Autodesk Fusion 360 part; units mm, degrees
(part 7 of 8)
  spline S32 degree 5 poles (-4.5955, -17.2194) (-4.5901, -17.2152) (-4.5794, -17.2068) (-4.5635, -17.1938) (-4.543, -17.1757) (-4.5182, -17.1521) (-4.4941, -17.1278) (-4.4703, -17.103) (-4.4466, -17.078) (-4.4232, -17.0528) (-4.3998, -17.0274) (-4.3767, -17.0018) (-4.3538, -16.9759) (-4.3312, -16.9497) (-4.3089, -16.9231) (-4.2869, -16.8962) (-4.2651, -16.869) (-4.2435, -16.8416) (-4.2221, -16.814) (-4.2009, -16.7862) (-4.1798, -16.7583) (-4.1589, -16.7301) (-4.1383, -16.7018) (-4.1177, -16.6732) (-4.0974, -16.6444) (-4.0773, -16.6154) (-4.0574, -16.5863) (-4.0376, -16.5569) (-4.018, -16.5274) (-3.9985, -16.4977) (-3.9792, -16.4679) (-3.9601, -16.4379) (-3.9411, -16.4077) (-3.9223, -16.3774) (-3.9037, -16.3469) (-3.8852, -16.3163) (-3.8668, -16.2855) (-3.8486, -16.2545) (-3.8306, -16.2234) (-3.8127, -16.1922) (-3.795, -16.1608) (-3.7774, -16.1293) (-3.76, -16.0976) (-3.7427, -16.0658) (-3.7255, -16.0339) (-3.7085, -16.0018) (-3.6917, -15.9696) (-3.6749, -15.9373) (-3.6584, -15.9048) (-3.6419, -15.8722) (-3.6256, -15.8395) (-3.6095, -15.8066) (-3.5935, -15.7737) (-3.5776, -15.7406) (-3.5619, -15.7073) (-3.5463, -15.674) (-3.5308, -15.6406) (-3.5155, -15.607) (-3.5003, -15.5733) (-3.4853, -15.5395) (-3.4704, -15.5056) (-3.4556, -15.4715) (-3.4409, -15.4374) (-3.4264, -15.4031) (-3.412, -15.3688) (-3.3978, -15.3343) (-3.3837, -15.2997) (-3.3697, -15.265) (-3.3559, -15.2302) (-3.3422, -15.1953) (-3.3286, -15.1603) (-3.3178, -15.1322) (-3.3098, -15.1111) (-3.3045, -15.097) (-3.3018, -15.09) knots 0 0 0 0 0 0 0.01428571 0.02857143 0.04285714 0.05714286 0.07142857 0.08571429 0.1 0.11428571 0.12857143 0.14285714 0.15714286 0.17142857 0.18571429 0.2 0.21428571 0.22857143 0.24285714 0.25714286 0.27142857 0.28571429 0.3 0.31428571 0.32857143 0.34285714 0.35714286 0.37142857 0.38571429 0.4 0.41428571 0.42857143 0.44285714 0.45714286 0.47142857 0.48571429 0.5 0.51428571 0.52857143 0.54285714 0.55714286 0.57142857 0.58571429 0.6 0.61428571 0.62857143 0.64285714 0.65714286 0.67142857 0.68571429 0.7 0.71428571 0.72857143 0.74285714 0.75714286 0.77142857 0.78571429 0.8 0.81428571 0.82857143 0.84285714 0.85714286 0.87142857 0.88571429 0.9 0.91428571 0.92857143 0.94285714 0.95714286 0.97142857 0.98571429 1 1 1 1 1 1
  arc A66 (-3.3018, -15.09) -> (-3.8891, -14.427) centre (-17.3506, -26.9445) ccw
  spline S33 degree 5 poles (-3.8891, -14.427) (-3.8965, -14.4288) (-3.9111, -14.4324) (-3.933, -14.4378) (-3.9622, -14.4451) (-3.9986, -14.4544) (-4.0349, -14.4638) (-4.0711, -14.4733) (-4.1072, -14.483) (-4.1432, -14.4929) (-4.1792, -14.5028) (-4.215, -14.513) (-4.2508, -14.5233) (-4.2864, -14.5337) (-4.322, -14.5442) (-4.3575, -14.555) (-4.3929, -14.5658) (-4.4281, -14.5768) (-4.4633, -14.588) (-4.4984, -14.5993) (-4.5334, -14.6108) (-4.5682, -14.6224) (-4.603, -14.6342) (-4.6377, -14.6461) (-4.6722, -14.6581) (-4.7067, -14.6704) (-4.741, -14.6828) (-4.7752, -14.6953) (-4.8093, -14.708) (-4.8434, -14.7208) (-4.8772, -14.7339) (-4.911, -14.747) (-4.9447, -14.7604) (-4.9782, -14.7739) (-5.0116, -14.7875) (-5.0449, -14.8013) (-5.0781, -14.8153) (-5.1111, -14.8295) (-5.144, -14.8438) (-5.1768, -14.8583) (-5.2095, -14.873) (-5.242, -14.8878) (-5.2744, -14.9028) (-5.3066, -14.918) (-5.3387, -14.9334) (-5.3706, -14.949) (-5.4024, -14.9647) (-5.4341, -14.9806) (-5.4656, -14.9967) (-5.497, -15.013) (-5.5281, -15.0295) (-5.5592, -15.0462) (-5.59, -15.0631) (-5.6206, -15.0802) (-5.6511, -15.0975) (-5.6814, -15.1151) (-5.7116, -15.1328) (-5.7415, -15.1507) (-5.7713, -15.1688) (-5.8009, -15.1872) (-5.8303, -15.2058) (-5.8593, -15.2247) (-5.8881, -15.244) (-5.9166, -15.2636) (-5.9448, -15.2835) (-5.9728, -15.3036) (-6.0007, -15.3239) (-6.0283, -15.3443) (-6.0558, -15.3649) (-6.0829, -15.386) (-6.1093, -15.4078) (-6.1297, -15.4259) (-6.1445, -15.4401) (-6.1542, -15.4498) (-6.159, -15.4546) knots -1 -1 -1 -1 -1 -1 -0.98571429 -0.97142857 -0.95714286 -0.94285714 -0.92857143 -0.91428571 -0.9 -0.88571429 -0.87142857 -0.85714286 -0.84285714 -0.82857143 -0.81428571 -0.8 -0.78571429 -0.77142857 -0.75714286 -0.74285714 -0.72857143 -0.71428571 -0.7 -0.68571429 -0.67142857 -0.65714286 -0.64285714 -0.62857143 -0.61428571 -0.6 -0.58571429 -0.57142857 -0.55714286 -0.54285714 -0.52857143 -0.51428571 -0.5 -0.48571429 -0.47142857 -0.45714286 -0.44285714 -0.42857143 -0.41428571 -0.4 -0.38571429 -0.37142857 -0.35714286 -0.34285714 -0.32857143 -0.31428571 -0.3 -0.28571429 -0.27142857 -0.25714286 -0.24285714 -0.22857143 -0.21428571 -0.2 -0.18571429 -0.17142857 -0.15714286 -0.14285714 -0.12857143 -0.11428571 -0.1 -0.08571429 -0.07142857 -0.05714286 -0.04285714 -0.02857143 -0.01428571 0 0 0 0 0 0
  line L33 (-6.159, -15.4546) -> (-6.2327, -15.5301)
  arc A67 (-6.9279, -15.5497) -> (-6.2327, -15.5301) centre (-6.5904, -15.1808) ccw
  arc A68 (-6.9279, -15.5497) -> (-7.2953, -15.2243) centre (-17.3506, -26.9445) ccw
  arc A69 (-7.3596, -14.5317) -> (-7.2953, -15.2243) centre (-6.9697, -14.8448) ccw
  line L34 (-7.3596, -14.5317) -> (-7.2936, -14.4495)
  spline S34 degree 5 poles (-7.2936, -14.4495) (-7.2893, -14.4442) (-7.2808, -14.4334) (-7.2686, -14.417) (-7.253, -14.3945) (-7.2346, -14.3657) (-7.2169, -14.3363) (-7.1997, -14.3065) (-7.1828, -14.2766) (-7.1661, -14.2465) (-7.1495, -14.2162) (-7.1331, -14.1858) (-7.1171, -14.1552) (-7.1014, -14.1243) (-7.0861, -14.0932) (-7.0712, -14.0618) (-7.0565, -14.0302) (-7.0422, -13.9985) (-7.028, -13.9665) (-7.014, -13.9345) (-7.0003, -13.9023) (-6.9867, -13.87) (-6.9734, -13.8375) (-6.9604, -13.8048) (-6.9475, -13.772) (-6.9349, -13.7391) (-6.9225, -13.706) (-6.9103, -13.6728) (-6.8984, -13.6394) (-6.8866, -13.6059) (-6.875, -13.5724) (-6.8636, -13.5386) (-6.8524, -13.5048) (-6.8414, -13.4709) (-6.8306, -13.4368) (-6.8199, -13.4026) (-6.8095, -13.3683) (-6.7993, -13.3339) (-6.7892, -13.2994) (-6.7793, -13.2648) (-6.7696, -13.2301) (-6.7601, -13.1953) (-6.7507, -13.1604) (-6.7415, -13.1253) (-6.7325, -13.0902) (-6.7237, -13.055) (-6.715, -13.0197) (-6.7065, -12.9843) (-6.6982, -12.9488) (-6.6901, -12.9132) (-6.6821, -12.8776) (-6.6743, -12.8418) (-6.6666, -12.806) (-6.6591, -12.77) (-6.6518, -12.734) (-6.6446, -12.6979) (-6.6376, -12.6617) (-6.6308, -12.6255) (-6.6241, -12.5891) (-6.6176, -12.5527) (-6.6112, -12.5162) (-6.605, -12.4796) (-6.599, -12.443) (-6.5931, -12.4062) (-6.5873, -12.3694) (-6.5818, -12.3325) (-6.5763, -12.2956) (-6.5711, -12.2585) (-6.5659, -12.2214) (-6.561, -12.1843) (-6.5562, -12.147) (-6.5524, -12.1172) (-6.5497, -12.0948) (-6.5479, -12.0798) (-6.547, -12.0723) knots 0 0 0 0 0 0 0.01428571 0.02857143 0.04285714 0.05714286 0.07142857 0.08571429 0.1 0.11428571 0.12857143 0.14285714 0.15714286 0.17142857 0.18571429 0.2 0.21428571 0.22857143 0.24285714 0.25714286 0.27142857 0.28571429 0.3 0.31428571 0.32857143 0.34285714 0.35714286 0.37142857 0.38571429 0.4 0.41428571 0.42857143 0.44285714 0.45714286 0.47142857 0.48571429 0.5 0.51428571 0.52857143 0.54285714 0.55714286 0.57142857 0.58571429 0.6 0.61428571 0.62857143 0.64285714 0.65714286 0.67142857 0.68571429 0.7 0.71428571 0.72857143 0.74285714 0.75714286 0.77142857 0.78571429 0.8 0.81428571 0.82857143 0.84285714 0.85714286 0.87142857 0.88571429 0.9 0.91428571 0.92857143 0.94285714 0.95714286 0.97142857 0.98571429 1 1 1 1 1 1
  arc A70 (-6.547, -12.0723) -> (-7.2759, -11.5692) centre (-17.3506, -26.9445) ccw
  spline S35 degree 5 poles (-7.2759, -11.5692) (-7.2826, -11.5727) (-7.296, -11.5797) (-7.3159, -11.5902) (-7.3425, -11.6043) (-7.3756, -11.622) (-7.4086, -11.6398) (-7.4415, -11.6577) (-7.4743, -11.6758) (-7.5069, -11.694) (-7.5394, -11.7122) (-7.5718, -11.7307) (-7.604, -11.7492) (-7.6362, -11.7678) (-7.6682, -11.7866) (-7.7, -11.8055) (-7.7318, -11.8245) (-7.7634, -11.8437) (-7.7949, -11.8629) (-7.8262, -11.8823) (-7.8575, -11.9018) (-7.8885, -11.9214) (-7.9195, -11.9412) (-7.9503, -11.961) (-7.9809, -11.981) (-8.0115, -12.0011) (-8.0418, -12.0214) (-8.0721, -12.0417) (-8.1022, -12.0622) (-8.1321, -12.0829) (-8.1619, -12.1036) (-8.1915, -12.1245) (-8.221, -12.1455) (-8.2504, -12.1666) (-8.2795, -12.1879) (-8.3085, -12.2093) (-8.3374, -12.2308) (-8.3661, -12.2524) (-8.3946, -12.2742) (-8.423, -12.2961) (-8.4512, -12.3182) (-8.4792, -12.3404) (-8.507, -12.3627) (-8.5347, -12.3852) (-8.5622, -12.4078) (-8.5895, -12.4305) (-8.6166, -12.4534) (-8.6435, -12.4764) (-8.6703, -12.4996) (-8.6968, -12.5229) (-8.7231, -12.5464) (-8.7493, -12.57) (-8.7751, -12.5938) (-8.8008, -12.6178) (-8.8262, -12.6419) (-8.8515, -12.6662) (-8.8765, -12.6906) (-8.9013, -12.7152) (-8.9259, -12.7399) (-8.9502, -12.7648) (-8.9743, -12.7899) (-8.998, -12.8152) (-9.0213, -12.8408) (-9.0443, -12.8667) (-9.0669, -12.8928) (-9.0893, -12.919) (-9.1115, -12.9453) (-9.1335, -12.9718) (-9.1552, -12.9984) (-9.1764, -13.0253) (-9.1968, -13.0528) (-9.2123, -13.0753) (-9.2233, -13.0926) (-9.2304, -13.1043) (-9.2339, -13.1102) knots -1 -1 -1 -1 -1 -1 -0.98571429 -0.97142857 -0.95714286 -0.94285714 -0.92857143 -0.91428571 -0.9 -0.88571429 -0.87142857 -0.85714286 -0.84285714 -0.82857143 -0.81428571 -0.8 -0.78571429 -0.77142857 -0.75714286 -0.74285714 -0.72857143 -0.71428571 -0.7 -0.68571429 -0.67142857 -0.65714286 -0.64285714 -0.62857143 -0.61428571 -0.6 -0.58571429 -0.57142857 -0.55714286 -0.54285714 -0.52857143 -0.51428571 -0.5 -0.48571429 -0.47142857 -0.45714286 -0.44285714 -0.42857143 -0.41428571 -0.4 -0.38571429 -0.37142857 -0.35714286 -0.34285714 -0.32857143 -0.31428571 -0.3 -0.28571429 -0.27142857 -0.25714286 -0.24285714 -0.22857143 -0.21428571 -0.2 -0.18571429 -0.17142857 -0.15714286 -0.14285714 -0.12857143 -0.11428571 -0.1 -0.08571429 -0.07142857 -0.05714286 -0.04285714 -0.02857143 -0.01428571 0 0 0 0 0 0
  line L35 (-9.2339, -13.1102) -> (-9.2874, -13.2011)
  arc A71 (-9.9577, -13.3865) -> (-9.2874, -13.2011) centre (-9.7183, -12.9475) ccw
  arc A72 (-9.9577, -13.3865) -> (-10.3923, -13.1584) centre (-17.3506, -26.9445) ccw
  arc A73 (-10.6205, -12.5014) -> (-10.3923, -13.1584) centre (-10.167, -12.7121) ccw
  line L36 (-10.6205, -12.5014) -> (-10.576, -12.4058)
  spline S36 degree 5 poles (-10.576, -12.4058) (-10.5732, -12.3996) (-10.5675, -12.3871) (-10.5596, -12.3682) (-10.5498, -12.3427) (-10.5389, -12.3103) (-10.5288, -12.2775) (-10.5192, -12.2445) (-10.5099, -12.2114) (-10.5008, -12.1781) (-10.492, -12.1448) (-10.4834, -12.1114) (-10.4751, -12.0778) (-10.4673, -12.0441) (-10.4599, -12.0102) (-10.4529, -11.9761) (-10.4463, -11.942) (-10.4399, -11.9077) (-10.4338, -11.8733) (-10.4279, -11.8388) (-10.4222, -11.8043) (-10.4168, -11.7696) (-10.4117, -11.7349) (-10.4068, -11.7001) (-10.4022, -11.6652) (-10.3978, -11.6302) (-10.3937, -11.5951) (-10.3899, -11.5599) (-10.3862, -11.5246) (-10.3828, -11.4893) (-10.3795, -11.4539) (-10.3765, -11.4185) (-10.3738, -11.383) (-10.3712, -11.3474) (-10.3689, -11.3117) (-10.3667, -11.276) (-10.3648, -11.2402) (-10.3631, -11.2043) (-10.3616, -11.1684) (-10.3602, -11.1324) (-10.3591, -11.0964) (-10.3582, -11.0603) (-10.3575, -11.0242) (-10.3569, -10.988) (-10.3566, -10.9517) (-10.3564, -10.9154) (-10.3565, -10.8791) (-10.3567, -10.8427) (-10.3571, -10.8062) (-10.3577, -10.7697) (-10.3585, -10.7332) (-10.3595, -10.6966) (-10.3606, -10.6599) (-10.362, -10.6233) (-10.3635, -10.5865) (-10.3651, -10.5498) (-10.367, -10.513) (-10.369, -10.4761) (-10.3713, -10.4392) (-10.3736, -10.4023) (-10.3762, -10.3653) (-10.3789, -10.3283) (-10.3818, -10.2913) (-10.3849, -10.2542) (-10.3881, -10.2171) (-10.3915, -10.18) (-10.3951, -10.1428) (-10.3989, -10.1056) (-10.4028, -10.0683) (-10.4069, -10.0311) (-10.4111, -9.9938) (-10.4146, -9.9639) (-10.4173, -9.9415) (-10.4192, -9.9265) (-10.4201, -9.919) knots 0 0 0 0 0 0 0.01428571 0.02857143 0.04285714 0.05714286 0.07142857 0.08571429 0.1 0.11428571 0.12857143 0.14285714 0.15714286 0.17142857 0.18571429 0.2 0.21428571 0.22857143 0.24285714 0.25714286 0.27142857 0.28571429 0.3 0.31428571 0.32857143 0.34285714 0.35714286 0.37142857 0.38571429 0.4 0.41428571 0.42857143 0.44285714 0.45714286 0.47142857 0.48571429 0.5 0.51428571 0.52857143 0.54285714 0.55714286 0.57142857 0.58571429 0.6 0.61428571 0.62857143 0.64285714 0.65714286 0.67142857 0.68571429 0.7 0.71428571 0.72857143 0.74285714 0.75714286 0.77142857 0.78571429 0.8 0.81428571 0.82857143 0.84285714 0.85714286 0.87142857 0.88571429 0.9 0.91428571 0.92857143 0.94285714 0.95714286 0.97142857 0.98571429 1 1 1 1 1 1
  arc A74 (-10.4201, -9.919) -> (-11.2482, -9.605) centre (-17.3506, -26.9445) ccw
  spline S37 degree 5 poles (-11.2482, -9.605) (-11.2539, -9.61) (-11.2652, -9.6199) (-11.2821, -9.6349) (-11.3045, -9.6549) (-11.3324, -9.68) (-11.3602, -9.7052) (-11.3878, -9.7305) (-11.4153, -9.7559) (-11.4426, -9.7813) (-11.4698, -9.8069) (-11.4968, -9.8325) (-11.5237, -9.8582) (-11.5505, -9.884) (-11.577, -9.9099) (-11.6035, -9.9359) (-11.6297, -9.962) (-11.6559, -9.9881) (-11.6818, -10.0143) (-11.7076, -10.0406) (-11.7333, -10.067) (-11.7587, -10.0935) (-11.7841, -10.1201) (-11.8092, -10.1468) (-11.8342, -10.1735) (-11.859, -10.2004) (-11.8837, -10.2273) (-11.9082, -10.2543) (-11.9325, -10.2814) (-11.9566, -10.3086) (-11.9806, -10.3358) (-12.0043, -10.3632) (-12.0279, -10.3906) (-12.0514, -10.4182) (-12.0746, -10.4458) (-12.0977, -10.4735) (-12.1205, -10.5013) (-12.1432, -10.5292) (-12.1657, -10.5572) (-12.188, -10.5853) (-12.2101, -10.6134) (-12.232, -10.6417) (-12.2537, -10.67) (-12.2751, -10.6984) (-12.2964, -10.727) (-12.3175, -10.7556) (-12.3383, -10.7843) (-12.359, -10.8131) (-12.3794, -10.842) (-12.3996, -10.871) (-12.4195, -10.9001) (-12.4392, -10.9293) (-12.4587, -10.9586) (-12.4778, -10.988) (-12.4968, -11.0175) (-12.5155, -11.0471) (-12.5339, -11.0768) (-12.5521, -11.1066) (-12.5701, -11.1365) (-12.5878, -11.1665) (-12.6051, -11.1966) (-12.622, -11.2269) (-12.6386, -11.2573) (-12.6547, -11.2879) (-12.6704, -11.3186) (-12.6858, -11.3495) (-12.7011, -11.3804) (-12.7161, -11.4113) (-12.7308, -11.4424) (-12.745, -11.4736) (-12.7583, -11.5051) (-12.7679, -11.5307) (-12.7745, -11.5501) (-12.7786, -11.5632) (-12.7805, -11.5697) knots -1 -1 -1 -1 -1 -1 -0.98571429 -0.97142857 -0.95714286 -0.94285714 -0.92857143 -0.91428571 -0.9 -0.88571429 -0.87142857 -0.85714286 -0.84285714 -0.82857143 -0.81428571 -0.8 -0.78571429 -0.77142857 -0.75714286 -0.74285714 -0.72857143 -0.71428571 -0.7 -0.68571429 -0.67142857 -0.65714286 -0.64285714 -0.62857143 -0.61428571 -0.6 -0.58571429 -0.57142857 -0.55714286 -0.54285714 -0.52857143 -0.51428571 -0.5 -0.48571429 -0.47142857 -0.45714286 -0.44285714 -0.42857143 -0.41428571 -0.4 -0.38571429 -0.37142857 -0.35714286 -0.34285714 -0.32857143 -0.31428571 -0.3 -0.28571429 -0.27142857 -0.25714286 -0.24285714 -0.22857143 -0.21428571 -0.2 -0.18571429 -0.17142857 -0.15714286 -0.14285714 -0.12857143 -0.11428571 -0.1 -0.08571429 -0.07142857 -0.05714286 -0.04285714 -0.02857143 -0.01428571 0 0 0 0 0 0
  line L37 (-12.7805, -11.5697) -> (-12.8107, -11.6708)
  arc A75 (-13.4171, -12.0112) -> (-12.8107, -11.6708) centre (-13.2898, -11.5277) ccw
  arc A76 (-13.4171, -12.0112) -> (-13.8937, -11.8938) centre (-17.3506, -26.9445) ccw
  arc A77 (-14.2725, -11.3105) -> (-13.8937, -11.8938) centre (-13.7818, -11.4065) ccw
  line L38 (-14.2725, -11.3105) -> (-14.2522, -11.207)
  spline S38 degree 5 poles (-14.2522, -11.207) (-14.2509, -11.2003) (-14.2485, -11.1868) (-14.2453, -11.1666) (-14.2419, -11.1394) (-14.239, -11.1054) (-14.237, -11.0711) (-14.2356, -11.0368) (-14.2346, -11.0024) (-14.2337, -10.968) (-14.2331, -10.9335) (-14.2327, -10.899) (-14.2328, -10.8644) (-14.2332, -10.8298) (-14.2342, -10.7951) (-14.2355, -10.7604) (-14.2372, -10.7256) (-14.2393, -10.6908) (-14.2415, -10.6559) (-14.2441, -10.6211) (-14.2469, -10.5862) (-14.2499, -10.5512) (-14.2532, -10.5163) (-14.2568, -10.4813) (-14.2607, -10.4463) (-14.2648, -10.4113) (-14.2692, -10.3762) (-14.2739, -10.3411) (-14.2788, -10.306) (-14.2839, -10.2709) (-14.2892, -10.2358) (-14.2948, -10.2006) (-14.3006, -10.1655) (-14.3067, -10.1303) (-14.3129, -10.0951) (-14.3194, -10.0599) (-14.3261, -10.0247) (-14.333, -9.9895) (-14.3401, -9.9542) (-14.3474, -9.919) (-14.355, -9.8837) (-14.3627, -9.8485) (-14.3707, -9.8132) (-14.3788, -9.778) (-14.3871, -9.7427) (-14.3957, -9.7074) (-14.4044, -9.6721) (-14.4134, -9.6368) (-14.4225, -9.6015) (-14.4318, -9.5662) (-14.4413, -9.5309) (-14.451, -9.4956) (-14.4609, -9.4603) (-14.471, -9.425) (-14.4812, -9.3897) (-14.4916, -9.3544) (-14.5023, -9.3192) (-14.513, -9.2839) (-14.524, -9.2486) (-14.5352, -9.2133) (-14.5465, -9.178) (-14.558, -9.1427) (-14.5697, -9.1075) (-14.5816, -9.0722) (-14.5936, -9.0369) (-14.6058, -9.0017) (-14.6182, -8.9665) (-14.6307, -8.9312) (-14.6434, -8.896) (-14.6563, -8.8608) (-14.6693, -8.8256) (-14.6799, -8.7974) (-14.6879, -8.7763) (-14.6933, -8.7622) (-14.696, -8.7552) knots 0 0 0 0 0 0 0.01428571 0.02857143 0.04285714 0.05714286 0.07142857 0.08571429 0.1 0.11428571 0.12857143 0.14285714 0.15714286 0.17142857 0.18571429 0.2 0.21428571 0.22857143 0.24285714 0.25714286 0.27142857 0.28571429 0.3 0.31428571 0.32857143 0.34285714 0.35714286 0.37142857 0.38571429 0.4 0.41428571 0.42857143 0.44285714 0.45714286 0.47142857 0.48571429 0.5 0.51428571 0.52857143 0.54285714 0.55714286 0.57142857 0.58571429 0.6 0.61428571 0.62857143 0.64285714 0.65714286 0.67142857 0.68571429 0.7 0.71428571 0.72857143 0.74285714 0.75714286 0.77142857 0.78571429 0.8 0.81428571 0.82857143 0.84285714 0.85714286 0.87142857 0.88571429 0.9 0.91428571 0.92857143 0.94285714 0.95714286 0.97142857 0.98571429 1 1 1 1 1 1
  arc A78 (-14.696, -8.7552) -> (-15.5752, -8.6484) centre (-17.3506, -26.9445) ccw
  spline S39 degree 5 poles (-15.5752, -8.6484) (-15.5795, -8.6546) (-15.588, -8.667) (-15.6009, -8.6856) (-15.6179, -8.7104) (-15.639, -8.7415) (-15.6599, -8.7726) (-15.6807, -8.8037) (-15.7013, -8.8349) (-15.7217, -8.8662) (-15.742, -8.8975) (-15.7621, -8.9289) (-15.7821, -8.9603) (-15.8018, -8.9917) (-15.8215, -9.0232) (-15.8409, -9.0547) (-15.8602, -9.0863) (-15.8793, -9.118) (-15.8982, -9.1497) (-15.9169, -9.1814) (-15.9355, -9.2132) (-15.9539, -9.245) (-15.9721, -9.2768) (-15.9902, -9.3087) (-16.008, -9.3407) (-16.0257, -9.3727) (-16.0432, -9.4047) (-16.0605, -9.4368) (-16.0776, -9.4689) (-16.0946, -9.5011) (-16.1113, -9.5333) (-16.1279, -9.5656) (-16.1442, -9.5979) (-16.1604, -9.6302) (-16.1763, -9.6626) (-16.1921, -9.695) (-16.2076, -9.7275) (-16.223, -9.76) (-16.2381, -9.7925) (-16.253, -9.8251) (-16.2677, -9.8578) (-16.2822, -9.8904) (-16.2965, -9.9231) (-16.3106, -9.9559) (-16.3244, -9.9887) (-16.338, -10.0215) (-16.3513, -10.0544) (-16.3645, -10.0873) (-16.3774, -10.1202) (-16.3901, -10.1532) (-16.4025, -10.1862) (-16.4146, -10.2193) (-16.4265, -10.2524) (-16.4381, -10.2855) (-16.4494, -10.3187) (-16.4604, -10.3519) (-16.4712, -10.3852) (-16.4818, -10.4185) (-16.4921, -10.4518) (-16.5021, -10.4852) (-16.5117, -10.5186) (-16.5209, -10.552) (-16.5297, -10.5855) (-16.538, -10.6191) (-16.5459, -10.6527) (-16.5535, -10.6863) (-16.5609, -10.7199) (-16.5681, -10.7536) (-16.575, -10.7872) (-16.5813, -10.8209) (-16.5866, -10.8548) (-16.5898, -10.8819) (-16.5916, -10.9023) (-16.5924, -10.916) (-16.5927, -10.9228) knots -1 -1 -1 -1 -1 -1 -0.98571429 -0.97142857 -0.95714286 -0.94285714 -0.92857143 -0.91428571 -0.9 -0.88571429 -0.87142857 -0.85714286 -0.84285714 -0.82857143 -0.81428571 -0.8 -0.78571429 -0.77142857 -0.75714286 -0.74285714 -0.72857143 -0.71428571 -0.7 -0.68571429 -0.67142857 -0.65714286 -0.64285714 -0.62857143 -0.61428571 -0.6 -0.58571429 -0.57142857 -0.55714286 -0.54285714 -0.52857143 -0.51428571 -0.5 -0.48571429 -0.47142857 -0.45714286 -0.44285714 -0.42857143 -0.41428571 -0.4 -0.38571429 -0.37142857 -0.35714286 -0.34285714 -0.32857143 -0.31428571 -0.3 -0.28571429 -0.27142857 -0.25714286 -0.24285714 -0.22857143 -0.21428571 -0.2 -0.18571429 -0.17142857 -0.15714286 -0.14285714 -0.12857143 -0.11428571 -0.1 -0.08571429 -0.07142857 -0.05714286 -0.04285714 -0.02857143 -0.01428571 0 0 0 0 0 0
  line L39 (-16.5927, -10.9228) -> (-16.5978, -11.0281)
  arc A79 (-17.1052, -11.5038) -> (-16.5978, -11.0281) centre (-17.0973, -11.0039) ccw
  arc A80 (-17.1052, -11.5038) -> (-17.596, -11.5038) centre (-17.3506, -26.9445) ccw
  arc A81 (-18.1034, -11.0281) -> (-17.596, -11.5038) centre (-17.604, -11.0039) ccw
  line L40 (-18.1034, -11.0281) -> (-18.1085, -10.9228)
  spline S40 degree 5 poles (-18.1085, -10.9228) (-18.1088, -10.916) (-18.1097, -10.9023) (-18.1114, -10.8819) (-18.1146, -10.8548) (-18.12, -10.8209) (-18.1262, -10.7872) (-18.1331, -10.7536) (-18.1403, -10.7199) (-18.1477, -10.6863) (-18.1553, -10.6527) (-18.1633, -10.6191) (-18.1716, -10.5855) (-18.1803, -10.552) (-18.1895, -10.5186) (-18.1992, -10.4852) (-18.2091, -10.4518) (-18.2194, -10.4185) (-18.23, -10.3852) (-18.2408, -10.3519) (-18.2518, -10.3187) (-18.2632, -10.2855) (-18.2747, -10.2524) (-18.2866, -10.2193) (-18.2988, -10.1862) (-18.3112, -10.1532) (-18.3238, -10.1202) (-18.3367, -10.0873) (-18.3499, -10.0544) (-18.3633, -10.0215) (-18.3769, -9.9887) (-18.3907, -9.9559) (-18.4047, -9.9231) (-18.419, -9.8904) (-18.4335, -9.8578) (-18.4482, -9.8251) (-18.4631, -9.7925) (-18.4783, -9.76) (-18.4936, -9.7275) (-18.5092, -9.695) (-18.5249, -9.6626) (-18.5409, -9.6302) (-18.557, -9.5979) (-18.5734, -9.5656) (-18.5899, -9.5333) (-18.6067, -9.5011) (-18.6236, -9.4689) (-18.6407, -9.4368) (-18.658, -9.4047) (-18.6755, -9.3727) (-18.6932, -9.3407) (-18.711, -9.3087) (-18.7291, -9.2768) (-18.7473, -9.245) (-18.7657, -9.2132) (-18.7843, -9.1814) (-18.803, -9.1497) (-18.822, -9.118) (-18.8411, -9.0863) (-18.8603, -9.0547) (-18.8798, -9.0232) (-18.8994, -8.9917) (-18.9192, -8.9603) (-18.9391, -8.9289) (-18.9592, -8.8975) (-18.9795, -8.8662) (-19, -8.8349) (-19.0206, -8.8037) (-19.0414, -8.7726) (-19.0623, -8.7415) (-19.0834, -8.7104) (-19.1004, -8.6856) (-19.1132, -8.667) (-19.1218, -8.6546) (-19.1261, -8.6484) knots 0 0 0 0 0 0 0.01428571 0.02857143 0.04285714 0.05714286 0.07142857 0.08571429 0.1 0.11428571 0.12857143 0.14285714 0.15714286 0.17142857 0.18571429 0.2 0.21428571 0.22857143 0.24285714 0.25714286 0.27142857 0.28571429 0.3 0.31428571 0.32857143 0.34285714 0.35714286 0.37142857 0.38571429 0.4 0.41428571 0.42857143 0.44285714 0.45714286 0.47142857 0.48571429 0.5 0.51428571 0.52857143 0.54285714 0.55714286 0.57142857 0.58571429 0.6 0.61428571 0.62857143 0.64285714 0.65714286 0.67142857 0.68571429 0.7 0.71428571 0.72857143 0.74285714 0.75714286 0.77142857 0.78571429 0.8 0.81428571 0.82857143 0.84285714 0.85714286 0.87142857 0.88571429 0.9 0.91428571 0.92857143 0.94285714 0.95714286 0.97142857 0.98571429 1 1 1 1 1 1
  arc A82 (-19.1261, -8.6484) -> (-20.0053, -8.7552) centre (-17.3506, -26.9445) ccw
  spline S41 degree 5 poles (-20.0053, -8.7552) (-20.008, -8.7622) (-20.0133, -8.7763) (-20.0213, -8.7974) (-20.0319, -8.8256) (-20.045, -8.8608) (-20.0578, -8.896) (-20.0705, -8.9312) (-20.0831, -8.9665) (-20.0955, -9.0017) (-20.1077, -9.0369) (-20.1197, -9.0722) (-20.1315, -9.1075) (-20.1432, -9.1427) (-20.1547, -9.178) (-20.1661, -9.2133) (-20.1772, -9.2486) (-20.1882, -9.2839) (-20.199, -9.3192) (-20.2096, -9.3544) (-20.22, -9.3897) (-20.2303, -9.425) (-20.2404, -9.4603) (-20.2502, -9.4956) (-20.2599, -9.5309) (-20.2694, -9.5662) (-20.2787, -9.6015) (-20.2879, -9.6368) (-20.2968, -9.6721) (-20.3055, -9.7074) (-20.3141, -9.7427) (-20.3224, -9.778) (-20.3306, -9.8132) (-20.3385, -9.8485) (-20.3463, -9.8837) (-20.3538, -9.919) (-20.3611, -9.9542) (-20.3682, -9.9895) (-20.3752, -10.0247) (-20.3819, -10.0599) (-20.3883, -10.0951) (-20.3946, -10.1303) (-20.4006, -10.1655) (-20.4064, -10.2006) (-20.412, -10.2358) (-20.4173, -10.2709) (-20.4225, -10.306) (-20.4273, -10.3411) (-20.432, -10.3762) (-20.4364, -10.4113) (-20.4406, -10.4463) (-20.4444, -10.4813) (-20.448, -10.5163) (-20.4513, -10.5512) (-20.4544, -10.5862) (-20.4572, -10.6211) (-20.4597, -10.6559) (-20.462, -10.6908) (-20.464, -10.7256) (-20.4657, -10.7604) (-20.4671, -10.7951) (-20.468, -10.8298) (-20.4685, -10.8644) (-20.4685, -10.899) (-20.4682, -10.9335) (-20.4675, -10.968) (-20.4667, -11.0024) (-20.4656, -11.0368) (-20.4642, -11.0711) (-20.4622, -11.1054) (-20.4593, -11.1394) (-20.456, -11.1666) (-20.4528, -11.1868) (-20.4503, -11.2003) (-20.449, -11.207) knots -1 -1 -1 -1 -1 -1 -0.98571429 -0.97142857 -0.95714286 -0.94285714 -0.92857143 -0.91428571 -0.9 -0.88571429 -0.87142857 -0.85714286 -0.84285714 -0.82857143 -0.81428571 -0.8 -0.78571429 -0.77142857 -0.75714286 -0.74285714 -0.72857143 -0.71428571 -0.7 -0.68571429 -0.67142857 -0.65714286 -0.64285714 -0.62857143 -0.61428571 -0.6 -0.58571429 -0.57142857 -0.55714286 -0.54285714 -0.52857143 -0.51428571 -0.5 -0.48571429 -0.47142857 -0.45714286 -0.44285714 -0.42857143 -0.41428571 -0.4 -0.38571429 -0.37142857 -0.35714286 -0.34285714 -0.32857143 -0.31428571 -0.3 -0.28571429 -0.27142857 -0.25714286 -0.24285714 -0.22857143 -0.21428571 -0.2 -0.18571429 -0.17142857 -0.15714286 -0.14285714 -0.12857143 -0.11428571 -0.1 -0.08571429 -0.07142857 -0.05714286 -0.04285714 -0.02857143 -0.01428571 0 0 0 0 0 0
  line L41 (-20.449, -11.207) -> (-20.4288, -11.3105)
  arc A83 (-20.8075, -11.8938) -> (-20.4288, -11.3105) centre (-20.9195, -11.4065) ccw
  arc A84 (-20.8075, -11.8938) -> (-21.2841, -12.0112) centre (-17.3506, -26.9445) ccw
  arc A85 (-21.8906, -11.6708) -> (-21.2841, -12.0112) centre (-21.4115, -11.5277) ccw
  line L42 (-21.8906, -11.6708) -> (-21.9207, -11.5697)
  spline S42 degree 5 poles (-21.9207, -11.5697) (-21.9227, -11.5632) (-21.9267, -11.5501) (-21.9333, -11.5307) (-21.943, -11.5051) (-21.9562, -11.4736) (-21.9704, -11.4424) (-21.9851, -11.4113) (-22.0001, -11.3804) (-22.0154, -11.3495) (-22.0308, -11.3186) (-22.0466, -11.2879) (-22.0627, -11.2573) (-22.0792, -11.2269) (-22.0961, -11.1966) (-22.1135, -11.1665) (-22.1312, -11.1365) (-22.1491, -11.1066) (-22.1673, -11.0768) (-22.1858, -11.0471) (-22.2045, -11.0175) (-22.2234, -10.988) (-22.2426, -10.9586) (-22.262, -10.9293) (-22.2817, -10.9001) (-22.3017, -10.871) (-22.3219, -10.842) (-22.3423, -10.8131) (-22.3629, -10.7843) (-22.3838, -10.7556) (-22.4048, -10.727) (-22.4261, -10.6984) (-22.4476, -10.67) (-22.4693, -10.6417) (-22.4912, -10.6134) (-22.5132, -10.5853) (-22.5355, -10.5572) (-22.558, -10.5292) (-22.5807, -10.5013) (-22.6036, -10.4735) (-22.6266, -10.4458) (-22.6499, -10.4182) (-22.6733, -10.3906) (-22.6969, -10.3632) (-22.7207, -10.3358) (-22.7446, -10.3086) (-22.7688, -10.2814) (-22.7931, -10.2543) (-22.8176, -10.2273) (-22.8422, -10.2004) (-22.867, -10.1735) (-22.892, -10.1468) (-22.9172, -10.1201) (-22.9425, -10.0935) (-22.968, -10.067) (-22.9936, -10.0406) (-23.0194, -10.0143) (-23.0454, -9.9881) (-23.0715, -9.962) (-23.0978, -9.9359) (-23.1242, -9.9099) (-23.1508, -9.884) (-23.1775, -9.8582) (-23.2044, -9.8325) (-23.2314, -9.8069) (-23.2586, -9.7813) (-23.2859, -9.7559) (-23.3134, -9.7305) (-23.341, -9.7052) (-23.3688, -9.68) (-23.3967, -9.6549) (-23.4192, -9.6349) (-23.4361, -9.6199) (-23.4474, -9.61) (-23.453, -9.605) knots 0 0 0 0 0 0 0.01428571 0.02857143 0.04285714 0.05714286 0.07142857 0.08571429 0.1 0.11428571 0.12857143 0.14285714 0.15714286 0.17142857 0.18571429 0.2 0.21428571 0.22857143 0.24285714 0.25714286 0.27142857 0.28571429 0.3 0.31428571 0.32857143 0.34285714 0.35714286 0.37142857 0.38571429 0.4 0.41428571 0.42857143 0.44285714 0.45714286 0.47142857 0.48571429 0.5 0.51428571 0.52857143 0.54285714 0.55714286 0.57142857 0.58571429 0.6 0.61428571 0.62857143 0.64285714 0.65714286 0.67142857 0.68571429 0.7 0.71428571 0.72857143 0.74285714 0.75714286 0.77142857 0.78571429 0.8 0.81428571 0.82857143 0.84285714 0.85714286 0.87142857 0.88571429 0.9 0.91428571 0.92857143 0.94285714 0.95714286 0.97142857 0.98571429 1 1 1 1 1 1
  arc A86 (-23.453, -9.605) -> (-24.2811, -9.919) centre (-17.3506, -26.9445) ccw
  spline S43 degree 5 poles (-24.2811, -9.919) (-24.2821, -9.9265) (-24.2839, -9.9415) (-24.2866, -9.9639) (-24.2901, -9.9938) (-24.2944, -10.0311) (-24.2985, -10.0683) (-24.3024, -10.1056) (-24.3061, -10.1428) (-24.3097, -10.18) (-24.3131, -10.2171) (-24.3163, -10.2542) (-24.3194, -10.2913) (-24.3223, -10.3283) (-24.325, -10.3653) (-24.3276, -10.4023) (-24.33, -10.4392) (-24.3322, -10.4761) (-24.3342, -10.513) (-24.3361, -10.5498) (-24.3378, -10.5865) (-24.3393, -10.6233) (-24.3406, -10.6599) (-24.3418, -10.6966) (-24.3427, -10.7332) (-24.3435, -10.7697) (-24.3441, -10.8062) (-24.3445, -10.8427) (-24.3447, -10.8791) (-24.3448, -10.9154) (-24.3446, -10.9517) (-24.3443, -10.988) (-24.3438, -11.0242) (-24.343, -11.0603) (-24.3421, -11.0964) (-24.341, -11.1324) (-24.3397, -11.1684) (-24.3382, -11.2043) (-24.3364, -11.2402) (-24.3345, -11.276) (-24.3324, -11.3117) (-24.33, -11.3474) (-24.3275, -11.383) (-24.3247, -11.4185) (-24.3217, -11.4539) (-24.3185, -11.4893) (-24.315, -11.5246) (-24.3114, -11.5599) (-24.3075, -11.5951) (-24.3034, -11.6302) (-24.299, -11.6652) (-24.2944, -11.7001) (-24.2896, -11.7349) (-24.2844, -11.7696) (-24.279, -11.8043) (-24.2734, -11.8388) (-24.2675, -11.8733) (-24.2613, -11.9077) (-24.255, -11.942) (-24.2483, -11.9761) (-24.2413, -12.0102) (-24.2339, -12.0441) (-24.2261, -12.0778) (-24.2179, -12.1114) (-24.2093, -12.1448) (-24.2004, -12.1781) (-24.1913, -12.2114) (-24.1821, -12.2445) (-24.1725, -12.2775) (-24.1624, -12.3103) (-24.1514, -12.3427) (-24.1416, -12.3682) (-24.1337, -12.3871) (-24.1281, -12.3996) (-24.1252, -12.4058) knots -1 -1 -1 -1 -1 -1 -0.98571429 -0.97142857 -0.95714286 -0.94285714 -0.92857143 -0.91428571 -0.9 -0.88571429 -0.87142857 -0.85714286 -0.84285714 -0.82857143 -0.81428571 -0.8 -0.78571429 -0.77142857 -0.75714286 -0.74285714 -0.72857143 -0.71428571 -0.7 -0.68571429 -0.67142857 -0.65714286 -0.64285714 -0.62857143 -0.61428571 -0.6 -0.58571429 -0.57142857 -0.55714286 -0.54285714 -0.52857143 -0.51428571 -0.5 -0.48571429 -0.47142857 -0.45714286 -0.44285714 -0.42857143 -0.41428571 -0.4 -0.38571429 -0.37142857 -0.35714286 -0.34285714 -0.32857143 -0.31428571 -0.3 -0.28571429 -0.27142857 -0.25714286 -0.24285714 -0.22857143 -0.21428571 -0.2 -0.18571429 -0.17142857 -0.15714286 -0.14285714 -0.12857143 -0.11428571 -0.1 -0.08571429 -0.07142857 -0.05714286 -0.04285714 -0.02857143 -0.01428571 0 0 0 0 0 0
  line L43 (-24.1252, -12.4058) -> (-24.0808, -12.5014)
  arc A87 (-24.3089, -13.1584) -> (-24.0808, -12.5014) centre (-24.5342, -12.7121) ccw
  arc A88 (-24.3089, -13.1584) -> (-24.7436, -13.3865) centre (-17.3506, -26.9445) ccw
  arc A89 (-25.4139, -13.2011) -> (-24.7436, -13.3865) centre (-24.9829, -12.9475) ccw
  line L44 (-25.4139, -13.2011) -> (-25.4673, -13.1102)
  spline S44 degree 5 poles (-25.4673, -13.1102) (-25.4708, -13.1043) (-25.4779, -13.0926) (-25.4889, -13.0753) (-25.5044, -13.0528) (-25.5248, -13.0253) (-25.5461, -12.9984) (-25.5678, -12.9718) (-25.5898, -12.9453) (-25.612, -12.919) (-25.6344, -12.8928) (-25.657, -12.8667) (-25.6799, -12.8408) (-25.7033, -12.8152) (-25.7269, -12.7899) (-25.751, -12.7648) (-25.7753, -12.7399) (-25.7999, -12.7152) (-25.8248, -12.6906) (-25.8498, -12.6662) (-25.875, -12.6419) (-25.9004, -12.6178) (-25.9261, -12.5938) (-25.952, -12.57) (-25.9781, -12.5464) (-26.0044, -12.5229) (-26.031, -12.4996) (-26.0577, -12.4764) (-26.0847, -12.4534) (-26.1118, -12.4305) (-26.1391, -12.4078) (-26.1665, -12.3852) (-26.1942, -12.3627) (-26.222, -12.3404) (-26.2501, -12.3182) (-26.2783, -12.2961) (-26.3066, -12.2742) (-26.3351, -12.2524) (-26.3638, -12.2308) (-26.3927, -12.2093) (-26.4217, -12.1879) (-26.4509, -12.1666) (-26.4802, -12.1455) (-26.5097, -12.1245) (-26.5393, -12.1036) (-26.5691, -12.0829) (-26.5991, -12.0622) (-26.6292, -12.0417) (-26.6594, -12.0214) (-26.6898, -12.0011) (-26.7203, -11.981) (-26.751, -11.961) (-26.7818, -11.9412) (-26.8127, -11.9214) (-26.8438, -11.9018) (-26.875, -11.8823) (-26.9063, -11.8629) (-26.9378, -11.8437) (-26.9694, -11.8245) (-27.0012, -11.8055) (-27.0331, -11.7866) (-27.0651, -11.7678) (-27.0972, -11.7492) (-27.1295, -11.7307) (-27.1618, -11.7122) (-27.1943, -11.694) (-27.227, -11.6758) (-27.2597, -11.6577) (-27.2926, -11.6398) (-27.3256, -11.622) (-27.3587, -11.6043) (-27.3853, -11.5902) (-27.4053, -11.5797) (-27.4186, -11.5727) (-27.4253, -11.5692) knots 0 0 0 0 0 0 0.01428571 0.02857143 0.04285714 0.05714286 0.07142857 0.08571429 0.1 0.11428571 0.12857143 0.14285714 0.15714286 0.17142857 0.18571429 0.2 0.21428571 0.22857143 0.24285714 0.25714286 0.27142857 0.28571429 0.3 0.31428571 0.32857143 0.34285714 0.35714286 0.37142857 0.38571429 0.4 0.41428571 0.42857143 0.44285714 0.45714286 0.47142857 0.48571429 0.5 0.51428571 0.52857143 0.54285714 0.55714286 0.57142857 0.58571429 0.6 0.61428571 0.62857143 0.64285714 0.65714286 0.67142857 0.68571429 0.7 0.71428571 0.72857143 0.74285714 0.75714286 0.77142857 0.78571429 0.8 0.81428571 0.82857143 0.84285714 0.85714286 0.87142857 0.88571429 0.9 0.91428571 0.92857143 0.94285714 0.95714286 0.97142857 0.98571429 1 1 1 1 1 1
  arc A90 (-27.4253, -11.5692) -> (-28.1542, -12.0723) centre (-17.3506, -26.9445) ccw
  spline S45 degree 5 poles (-28.1542, -12.0723) (-28.1533, -12.0798) (-28.1515, -12.0948) (-28.1488, -12.1172) (-28.1451, -12.147) (-28.1403, -12.1843) (-28.1353, -12.2214) (-28.1302, -12.2585) (-28.1249, -12.2956) (-28.1195, -12.3325) (-28.1139, -12.3694) (-28.1082, -12.4062) (-28.1023, -12.443) (-28.0962, -12.4796) (-28.09, -12.5162) (-28.0837, -12.5527) (-28.0771, -12.5891) (-28.0705, -12.6255) (-28.0636, -12.6617) (-28.0566, -12.6979) (-28.0495, -12.734) (-28.0421, -12.77) (-28.0346, -12.806) (-28.027, -12.8418) (-28.0192, -12.8776) (-28.0112, -12.9132) (-28.003, -12.9488) (-27.9947, -12.9843) (-27.9862, -13.0197) (-27.9776, -13.055) (-27.9687, -13.0902) (-27.9597, -13.1253) (-27.9505, -13.1604) (-27.9412, -13.1953) (-27.9317, -13.2301) (-27.9219, -13.2648) (-27.9121, -13.2994) (-27.902, -13.3339) (-27.8917, -13.3683) (-27.8813, -13.4026) (-27.8707, -13.4368) (-27.8599, -13.4709) (-27.8489, -13.5048) (-27.8377, -13.5386) (-27.8263, -13.5724) (-27.8147, -13.6059) (-27.8029, -13.6394) (-27.7909, -13.6728) (-27.7787, -13.706) (-27.7663, -13.7391) (-27.7537, -13.772) (-27.7409, -13.8048) (-27.7278, -13.8375) (-27.7145, -13.87) (-27.701, -13.9023) (-27.6872, -13.9345) (-27.6732, -13.9665) (-27.6591, -13.9985) (-27.6447, -14.0302) (-27.63, -14.0618) (-27.6151, -14.0932) (-27.5998, -14.1243) (-27.5841, -14.1552) (-27.5681, -14.1858) (-27.5518, -14.2162) (-27.5352, -14.2465) (-27.5184, -14.2766) (-27.5015, -14.3065) (-27.4843, -14.3363) (-27.4666, -14.3657) (-27.4482, -14.3945) (-27.4326, -14.417) (-27.4204, -14.4334) (-27.412, -14.4442) (-27.4077, -14.4495) knots -1 -1 -1 -1 -1 -1 -0.98571429 -0.97142857 -0.95714286 -0.94285714 -0.92857143 -0.91428571 -0.9 -0.88571429 -0.87142857 -0.85714286 -0.84285714 -0.82857143 -0.81428571 -0.8 -0.78571429 -0.77142857 -0.75714286 -0.74285714 -0.72857143 -0.71428571 -0.7 -0.68571429 -0.67142857 -0.65714286 -0.64285714 -0.62857143 -0.61428571 -0.6 -0.58571429 -0.57142857 -0.55714286 -0.54285714 -0.52857143 -0.51428571 -0.5 -0.48571429 -0.47142857 -0.45714286 -0.44285714 -0.42857143 -0.41428571 -0.4 -0.38571429 -0.37142857 -0.35714286 -0.34285714 -0.32857143 -0.31428571 -0.3 -0.28571429 -0.27142857 -0.25714286 -0.24285714 -0.22857143 -0.21428571 -0.2 -0.18571429 -0.17142857 -0.15714286 -0.14285714 -0.12857143 -0.11428571 -0.1 -0.08571429 -0.07142857 -0.05714286 -0.04285714 -0.02857143 -0.01428571 0 0 0 0 0 0
  line L45 (-27.4077, -14.4495) -> (-27.3417, -14.5317)
  arc A91 (-27.406, -15.2243) -> (-27.3417, -14.5317) centre (-27.7315, -14.8448) ccw
  arc A92 (-27.406, -15.2243) -> (-27.7734, -15.5497) centre (-17.3506, -26.9445) ccw
  arc A93 (-28.4686, -15.5301) -> (-27.7734, -15.5497) centre (-28.1108, -15.1808) ccw
  line L46 (-28.4686, -15.5301) -> (-28.5423, -15.4546)
  spline S46 degree 5 poles (-28.5423, -15.4546) (-28.547, -15.4498) (-28.5567, -15.4401) (-28.5715, -15.4259) (-28.592, -15.4078) (-28.6184, -15.386) (-28.6454, -15.3649) (-28.6729, -15.3443) (-28.7006, -15.3239) (-28.7284, -15.3036) (-28.7564, -15.2835) (-28.7847, -15.2636) (-28.8131, -15.244) (-28.8419, -15.2247) (-28.871, -15.2058) (-28.9003, -15.1872) (-28.9299, -15.1688) (-28.9597, -15.1507) (-28.9897, -15.1328) (-29.0198, -15.1151) (-29.0501, -15.0975) (-29.0806, -15.0802) (-29.1112, -15.0631) (-29.1421, -15.0462) (-29.1731, -15.0295) (-29.2043, -15.013) (-29.2356, -14.9967) (-29.2671, -14.9806) (-29.2988, -14.9647) (-29.3306, -14.949) (-29.3626, -14.9334) (-29.3946, -14.918) (-29.4269, -14.9028) (-29.4593, -14.8878) (-29.4918, -14.873) (-29.5244, -14.8583) (-29.5572, -14.8438) (-29.5901, -14.8295) (-29.6232, -14.8153) (-29.6563, -14.8013) (-29.6896, -14.7875) (-29.723, -14.7739) (-29.7566, -14.7604) (-29.7902, -14.747) (-29.824, -14.7339) (-29.8579, -14.7208) (-29.8919, -14.708) (-29.926, -14.6953) (-29.9602, -14.6828) (-29.9946, -14.6704) (-30.029, -14.6581) (-30.0636, -14.6461) (-30.0982, -14.6342) (-30.133, -14.6224) (-30.1679, -14.6108) (-30.2029, -14.5993) (-30.2379, -14.588) (-30.2731, -14.5768) (-30.3084, -14.5658) (-30.3438, -14.555) (-30.3792, -14.5442) (-30.4148, -14.5337) (-30.4505, -14.5233) (-30.4862, -14.513) (-30.5221, -14.5028) (-30.558, -14.4929) (-30.594, -14.483) (-30.6302, -14.4733) (-30.6664, -14.4638) (-30.7027, -14.4544) (-30.739, -14.4451) (-30.7682, -14.4378) (-30.7901, -14.4324) (-30.8048, -14.4288) (-30.8121, -14.427) knots 0 0 0 0 0 0 0.01428571 0.02857143 0.04285714 0.05714286 0.07142857 0.08571429 0.1 0.11428571 0.12857143 0.14285714 0.15714286 0.17142857 0.18571429 0.2 0.21428571 0.22857143 0.24285714 0.25714286 0.27142857 0.28571429 0.3 0.31428571 0.32857143 0.34285714 0.35714286 0.37142857 0.38571429 0.4 0.41428571 0.42857143 0.44285714 0.45714286 0.47142857 0.48571429 0.5 0.51428571 0.52857143 0.54285714 0.55714286 0.57142857 0.58571429 0.6 0.61428571 0.62857143 0.64285714 0.65714286 0.67142857 0.68571429 0.7 0.71428571 0.72857143 0.74285714 0.75714286 0.77142857 0.78571429 0.8 0.81428571 0.82857143 0.84285714 0.85714286 0.87142857 0.88571429 0.9 0.91428571 0.92857143 0.94285714 0.95714286 0.97142857 0.98571429 1 1 1 1 1 1
  arc A94 (-30.8121, -14.427) -> (-31.3994, -15.09) centre (-17.3506, -26.9445) ccw
  spline S47 degree 5 poles (-31.3994, -15.09) (-31.3967, -15.097) (-31.3914, -15.1111) (-31.3834, -15.1322) (-31.3727, -15.1603) (-31.3591, -15.1953) (-31.3454, -15.2302) (-31.3315, -15.265) (-31.3175, -15.2997) (-31.3034, -15.3343) (-31.2892, -15.3688) (-31.2748, -15.4031) (-31.2603, -15.4374) (-31.2457, -15.4715) (-31.2309, -15.5056) (-31.216, -15.5395) (-31.2009, -15.5733) (-31.1857, -15.607) (-31.1704, -15.6406) (-31.155, -15.674) (-31.1394, -15.7073) (-31.1236, -15.7406) (-31.1078, -15.7737) (-31.0917, -15.8066) (-31.0756, -15.8395) (-31.0593, -15.8722) (-31.0429, -15.9048) (-31.0263, -15.9373) (-31.0096, -15.9696) (-30.9927, -16.0018) (-30.9757, -16.0339) (-30.9586, -16.0658) (-30.9413, -16.0976) (-30.9238, -16.1293) (-30.9063, -16.1608) (-30.8885, -16.1922) (-30.8706, -16.2234) (-30.8526, -16.2545) (-30.8344, -16.2855) (-30.8161, -16.3163) (-30.7976, -16.3469) (-30.7789, -16.3774) (-30.7601, -16.4077) (-30.7411, -16.4379) (-30.722, -16.4679) (-30.7027, -16.4977) (-30.6833, -16.5274) (-30.6637, -16.5569) (-30.6439, -16.5863) (-30.6239, -16.6154) (-30.6038, -16.6444) (-30.5835, -16.6732) (-30.563, -16.7018) (-30.5423, -16.7301) (-30.5214, -16.7583) (-30.5003, -16.7862) (-30.4791, -16.814) (-30.4577, -16.8416) (-30.4361, -16.869) (-30.4144, -16.8962) (-30.3923, -16.9231) (-30.37, -16.9497) (-30.3474, -16.9759) (-30.3245, -17.0018) (-30.3014, -17.0274) (-30.2781, -17.0528) (-30.2546, -17.078) (-30.231, -17.103) (-30.2072, -17.1278) (-30.183, -17.1521) (-30.1582, -17.1757) (-30.1377, -17.1938) (-30.1219, -17.2068) (-30.1111, -17.2152) (-30.1057, -17.2194) knots -1 -1 -1 -1 -1 -1 -0.98571429 -0.97142857 -0.95714286 -0.94285714 -0.92857143 -0.91428571 -0.9 -0.88571429 -0.87142857 -0.85714286 -0.84285714 -0.82857143 -0.81428571 -0.8 -0.78571429 -0.77142857 -0.75714286 -0.74285714 -0.72857143 -0.71428571 -0.7 -0.68571429 -0.67142857 -0.65714286 -0.64285714 -0.62857143 -0.61428571 -0.6 -0.58571429 -0.57142857 -0.55714286 -0.54285714 -0.52857143 -0.51428571 -0.5 -0.48571429 -0.47142857 -0.45714286 -0.44285714 -0.42857143 -0.41428571 -0.4 -0.38571429 -0.37142857 -0.35714286 -0.34285714 -0.32857143 -0.31428571 -0.3 -0.28571429 -0.27142857 -0.25714286 -0.24285714 -0.22857143 -0.21428571 -0.2 -0.18571429 -0.17142857 -0.15714286 -0.14285714 -0.12857143 -0.11428571 -0.1 -0.08571429 -0.07142857 -0.05714286 -0.04285714 -0.02857143 -0.01428571 0 0 0 0 0 0
  line L47 (-30.1057, -17.2194) -> (-30.0219, -17.2834)
  arc A95 (-29.9186, -17.9712) -> (-30.0219, -17.2834) centre (-30.3255, -17.6807) ccw
  arc A96 (-29.9186, -17.9712) -> (-30.1974, -18.3752) centre (-17.3506, -26.9445) ccw
  arc A97 (-30.8771, -18.5225) -> (-30.1974, -18.3752) centre (-30.6134, -18.0977) ccw
  line L48 (-30.8771, -18.5225) -> (-30.9667, -18.4669)
  spline S48 degree 5 poles (-30.9667, -18.4669) (-30.9726, -18.4632) (-30.9843, -18.4562) (-31.002, -18.446) (-31.0262, -18.4333) (-31.0571, -18.4184) (-31.0884, -18.4045) (-31.12, -18.391) (-31.1518, -18.3778) (-31.1837, -18.3648) (-31.2157, -18.3519) (-31.2478, -18.3394) (-31.2802, -18.3272) (-31.3127, -18.3153) (-31.3455, -18.3039) (-31.3784, -18.2928) (-31.4115, -18.2821) (-31.4448, -18.2717) (-31.4782, -18.2614) (-31.5117, -18.2514) (-31.5453, -18.2417) (-31.5791, -18.2321) (-31.6129, -18.2228) (-31.6469, -18.2138) (-31.681, -18.205) (-31.7152, -18.1965) (-31.7496, -18.1882) (-31.784, -18.1801) (-31.8186, -18.1722) (-31.8532, -18.1645) (-31.888, -18.1571) (-31.9228, -18.1498) (-31.9577, -18.1428) (-31.9928, -18.1359) (-32.0279, -18.1293) (-32.0631, -18.1229) (-32.0984, -18.1167) (-32.1338, -18.1106) (-32.1692, -18.1048) (-32.2048, -18.0991) (-32.2404, -18.0937) (-32.2761, -18.0884) (-32.3119, -18.0833) (-32.3478, -18.0785) (-32.3837, -18.0737) (-32.4198, -18.0692) (-32.4558, -18.0649) (-32.492, -18.0607) (-32.5282, -18.0567) (-32.5646, -18.0529) (-32.6009, -18.0493) (-32.6374, -18.0459) (-32.6739, -18.0426) (-32.7104, -18.0395) (-32.7471, -18.0365) (-32.7838, -18.0338) (-32.8206, -18.0312) (-32.8574, -18.0288) (-32.8943, -18.0265) (-32.9312, -18.0244) (-32.9682, -18.0225) (-33.0053, -18.0208) (-33.0424, -18.0192) (-33.0796, -18.0178) (-33.1168, -18.0165) (-33.1541, -18.0154) (-33.1914, -18.0145) (-33.2288, -18.0137) (-33.2663, -18.0131) (-33.3038, -18.0127) (-33.3413, -18.0124) (-33.3714, -18.0123) (-33.394, -18.0123) (-33.409, -18.0123) (-33.4166, -18.0123) knots 0 0 0 0 0 0 0.01428571 0.02857143 0.04285714 0.05714286 0.07142857 0.08571429 0.1 0.11428571 0.12857143 0.14285714 0.15714286 0.17142857 0.18571429 0.2 0.21428571 0.22857143 0.24285714 0.25714286 0.27142857 0.28571429 0.3 0.31428571 0.32857143 0.34285714 0.35714286 0.37142857 0.38571429 0.4 0.41428571 0.42857143 0.44285714 0.45714286 0.47142857 0.48571429 0.5 0.51428571 0.52857143 0.54285714 0.55714286 0.57142857 0.58571429 0.6 0.61428571 0.62857143 0.64285714 0.65714286 0.67142857 0.68571429 0.7 0.71428571 0.72857143 0.74285714 0.75714286 0.77142857 0.78571429 0.8 0.81428571 0.82857143 0.84285714 0.85714286 0.87142857 0.88571429 0.9 0.91428571 0.92857143 0.94285714 0.95714286 0.97142857 0.98571429 1 1 1 1 1 1
  arc A98 (-33.4166, -18.0123) -> (-33.8281, -18.7965) centre (-17.3506, -26.9445) ccw
  spline S49 degree 5 poles (-33.8281, -18.7965) (-33.8239, -18.8027) (-33.8153, -18.8152) (-33.8025, -18.8337) (-33.7853, -18.8584) (-33.7638, -18.8892) (-33.7421, -18.9198) (-33.7203, -18.9502) (-33.6985, -18.9806) (-33.6765, -19.0108) (-33.6544, -19.0408) (-33.6322, -19.0708) (-33.6099, -19.1006) (-33.5876, -19.1302) (-33.5651, -19.1597) (-33.5425, -19.1891) (-33.5198, -19.2183) (-33.497, -19.2474) (-33.474, -19.2763) (-33.451, -19.3051) (-33.4279, -19.3337) (-33.4047, -19.3622) (-33.3814, -19.3906) (-33.3579, -19.4187) (-33.3344, -19.4468) (-33.3107, -19.4746) (-33.287, -19.5024) (-33.2631, -19.5299) (-33.2391, -19.5573) (-33.2151, -19.5846) (-33.1909, -19.6116) (-33.1666, -19.6385) (-33.1422, -19.6653) (-33.1177, -19.6918) (-33.0931, -19.7182) (-33.0683, -19.7445) (-33.0435, -19.7705) (-33.0185, -19.7964) (-32.9935, -19.8221) (-32.9683, -19.8476) (-32.943, -19.8729) (-32.9176, -19.8981) (-32.8921, -19.923) (-32.8664, -19.9478) (-32.8407, -19.9723) (-32.8148, -19.9967) (-32.7888, -20.0208) (-32.7627, -20.0448) (-32.7365, -20.0685) (-32.7101, -20.0921) (-32.6837, -20.1154) (-32.657, -20.1385) (-32.6303, -20.1613) (-32.6034, -20.1839) (-32.5764, -20.2062) (-32.5493, -20.2284) (-32.522, -20.2503) (-32.4946, -20.2719) (-32.4671, -20.2934) (-32.4395, -20.3145) (-32.4117, -20.3354) (-32.3836, -20.3558) (-32.3554, -20.3759) (-32.327, -20.3956) (-32.2984, -20.4149) (-32.2697, -20.434) (-32.2408, -20.4528) (-32.2119, -20.4715) (-32.1829, -20.4898) (-32.1536, -20.5076) (-32.1239, -20.5246) (-32.0996, -20.5373) (-32.0812, -20.5461) (-32.0687, -20.5517) (-32.0624, -20.5545) knots -1 -1 -1 -1 -1 -1 -0.98571429 -0.97142857 -0.95714286 -0.94285714 -0.92857143 -0.91428571 -0.9 -0.88571429 -0.87142857 -0.85714286 -0.84285714 -0.82857143 -0.81428571 -0.8 -0.78571429 -0.77142857 -0.75714286 -0.74285714 -0.72857143 -0.71428571 -0.7 -0.68571429 -0.67142857 -0.65714286 -0.64285714 -0.62857143 -0.61428571 -0.6 -0.58571429 -0.57142857 -0.55714286 -0.54285714 -0.52857143 -0.51428571 -0.5 -0.48571429 -0.47142857 -0.45714286 -0.44285714 -0.42857143 -0.41428571 -0.4 -0.38571429 -0.37142857 -0.35714286 -0.34285714 -0.32857143 -0.31428571 -0.3 -0.28571429 -0.27142857 -0.25714286 -0.24285714 -0.22857143 -0.21428571 -0.2 -0.18571429 -0.17142857 -0.15714286 -0.14285714 -0.12857143 -0.11428571 -0.1 -0.08571429 -0.07142857 -0.05714286 -0.04285714 -0.02857143 -0.01428571 0 0 0 0 0 0
  line L49 (-32.0624, -20.5545) -> (-31.9657, -20.5966)
  arc A99 (-31.7009, -21.2397) -> (-31.9657, -20.5966) centre (-32.1655, -21.055) ccw
  arc A100 (-31.7009, -21.2397) -> (-31.8749, -21.6986) centre (-17.3506, -26.9445) ccw
  arc A101 (-32.4996, -22.0043) -> (-31.8749, -21.6986) centre (-32.3452, -21.5288) ccw
  line L50 (-32.4996, -22.0043) -> (-32.5999, -21.9718)
  spline S50 degree 5 poles (-32.5999, -21.9718) (-32.6064, -21.9696) (-32.6195, -21.9656) (-32.6392, -21.9599) (-32.6657, -21.9534) (-32.6992, -21.9464) (-32.733, -21.9403) (-32.7669, -21.9347) (-32.8009, -21.9295) (-32.835, -21.9245) (-32.8691, -21.9198) (-32.9033, -21.9153) (-32.9376, -21.9111) (-32.9721, -21.9074) (-33.0066, -21.9042) (-33.0413, -21.9013) (-33.076, -21.8988) (-33.1108, -21.8966) (-33.1457, -21.8947) (-33.1806, -21.893) (-33.2156, -21.8916) (-33.2506, -21.8904) (-33.2857, -21.8895) (-33.3209, -21.8888) (-33.3561, -21.8884) (-33.3914, -21.8883) (-33.4267, -21.8885) (-33.4621, -21.8889) (-33.4975, -21.8895) (-33.533, -21.8904) (-33.5685, -21.8914) (-33.6041, -21.8927) (-33.6397, -21.8942) (-33.6753, -21.896) (-33.711, -21.898) (-33.7467, -21.9001) (-33.7825, -21.9026) (-33.8183, -21.9052) (-33.8541, -21.908) (-33.89, -21.911) (-33.9259, -21.9142) (-33.9618, -21.9177) (-33.9978, -21.9213) (-34.0338, -21.9251) (-34.0698, -21.9292) (-34.1059, -21.9334) (-34.1419, -21.9378) (-34.1781, -21.9424) (-34.2142, -21.9472) (-34.2504, -21.9522) (-34.2865, -21.9574) (-34.3227, -21.9628) (-34.359, -21.9683) (-34.3952, -21.9741) (-34.4315, -21.98) (-34.4678, -21.9861) (-34.5041, -21.9924) (-34.5404, -21.9989) (-34.5768, -22.0055) (-34.6132, -22.0123) (-34.6496, -22.0193) (-34.686, -22.0265) (-34.7224, -22.0338) (-34.7588, -22.0413) (-34.7953, -22.049) (-34.8317, -22.0569) (-34.8682, -22.0649) (-34.9047, -22.0731) (-34.9412, -22.0815) (-34.9777, -22.09) (-35.0142, -22.0988) (-35.0435, -22.1058) (-35.0654, -22.1112) (-35.08, -22.1149) (-35.0873, -22.1167) knots 0 0 0 0 0 0 0.01428571 0.02857143 0.04285714 0.05714286 0.07142857 0.08571429 0.1 0.11428571 0.12857143 0.14285714 0.15714286 0.17142857 0.18571429 0.2 0.21428571 0.22857143 0.24285714 0.25714286 0.27142857 0.28571429 0.3 0.31428571 0.32857143 0.34285714 0.35714286 0.37142857 0.38571429 0.4 0.41428571 0.42857143 0.44285714 0.45714286 0.47142857 0.48571429 0.5 0.51428571 0.52857143 0.54285714 0.55714286 0.57142857 0.58571429 0.6 0.61428571 0.62857143 0.64285714 0.65714286 0.67142857 0.68571429 0.7 0.71428571 0.72857143 0.74285714 0.75714286 0.77142857 0.78571429 0.8 0.81428571 0.82857143 0.84285714 0.85714286 0.87142857 0.88571429 0.9 0.91428571 0.92857143 0.94285714 0.95714286 0.97142857 0.98571429 1 1 1 1 1 1
  arc A102 (-35.0873, -22.1167) -> (-35.2993, -22.9766) centre (-17.3506, -26.9445) ccw